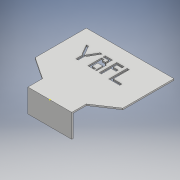
# Autodesk Inventor part: Body Front
Saved by Autodesk Inventor 2018 (Build 220112000, 112)
## iProperties
Created: 2018-04-26
Part Number: Body Front
Material: Generic
Document SubType Name: Modeling
Designer: HP
Density: 1 g/cm^3
Appearance: Default
Author: HP
Autodesk Inventor part; units mm, degrees
ref_plane "YZ Plane" through (0, 0, 0) normal (1, 0, 0) x (0, 1, 0)
ref_plane "XZ Plane" through (0, 0, 0) normal (0, 1, 0) x (-1, 0, 0)
ref_plane "XY Plane" through (0, 0, 0) normal (0, 0, 1) x (1, 0, 0)
sketch "Sketch1" plane through (0, 0, 0) normal (0, 0, 1) x (1, 0, 0)
  line L0 (-30, 0) -> (30, 0)
  line L1 (30, 0) -> (30, 20)
  line L2 (-30, 20) -> (-30, 0)
  line L3 (60, 40) -> (60, 110)
  line L4 (60, 110) -> (-60, 110)
  line L5 (-60, 110) -> (-60, 40)
  line L6 (-60, 40) -> (-30, 20)
  line L7 (30, 20) -> (60, 40)
  point P0 (0, 0)
  dimension "d0" = 60
  dimension "d1" = 20
  dimension "d2" = 120
  dimension "d3" = 70
  constraints: 16 end point, 2 parallel, 1 horizontal, 1 perpendicular
  measures "d0" distance of L2.start L1.end
  measures "d1" distance of L1.end L0.end
  measures "d2" distance of L4.end L3.end
  measures "d3" distance of L3.end L3.start
extrude "Extrusion1" add sketch "Sketch1" along normal blind 2
sketch "Sketch2" plane through (-30, 0, 0) normal (0, -1, 0) x (1, 0, 0)
  line L0 (60, 0) -> (60, 2) projected
  line L1 (60, 0) -> (0, 0)
  line L2 (0, 0) -> (0, -30)
  line L3 (0, -30) -> (60, -30)
  line L4 (60, -30) -> (60, 0)
  point P0 (30, 0)
  dimension "d6" = 60
  dimension "d7" = 30
  constraints: 8 end point, 2 parallel, 1 horizontal, 1 perpendicular
  measures "d6" distance of L3.end L2.end
  measures "d7" distance of L2.end L1.end
extrude "Extrusion2" add sketch "Sketch2" against normal blind 2
sketch "Sketch3" plane through (0, 0, 2) normal (0, 0, 1) x (1, 0, 0)
  line L0 (-37, 90) -> (-29.0967, 76.3111)
  line L1 (-37, 90) -> (-21.1935, 90) construction
  line L2 (-30.5967, 76.3111) -> (-32.0967, 76.3111)
  line L3 (-32.0967, 76.3111) -> (-39.25, 88.701)
  line L4 (-39.25, 88.701) -> (-40, 90)
  line L5 (-40, 90) -> (-37, 90)
  line L6 (-29.0967, 76.3111) -> (-21.1935, 90)
  line L7 (-21.1935, 90) -> (-18.1935, 90)
  line L8 (-18.1935, 90) -> (-26.0967, 76.3111)
  line L9 (-26.0967, 76.3111) -> (-27.5967, 76.3111)
  line L10 (-30.5967, 76.3111) -> (-30.5967, 66.3111)
  line L11 (-30.5967, 66.3111) -> (-27.5967, 66.3111)
  line L12 (-27.5967, 66.3111) -> (-27.5967, 76.3111)
  line L13 (-14.1935, 90) -> (-14.1935, 66.3111)
  line L14 (-14.1935, 90) -> (-4.1935, 90)
  line L15 (-4.1935, 90) -> (-4.1935, 79.933)
  line L16 (-4.1935, 79.933) -> (-2.1935, 79.933)
  line L17 (-2.1935, 79.933) -> (-2.1935, 66.3111)
  line L18 (-2.1935, 66.3111) -> (-14.1935, 66.3111)
  line L19 (-10.757, 87) -> (-10.757, 82.506)
  line L20 (-10.757, 82.506) -> (-6.2868, 82.506)
  line L21 (-6.2868, 82.506) -> (-6.2868, 87)
  line L22 (-6.2868, 87) -> (-10.757, 87)
  line L23 (-10.757, 76.3111) -> (-10.757, 68.4995)
  line L24 (-10.757, 68.4995) -> (-3.7569, 68.4995)
  line L25 (-3.7569, 68.4995) -> (-3.7569, 76.3111)
  line L26 (-3.7569, 76.3111) -> (-10.757, 76.3111)
  line L27 (1.8065, 65.8916) -> (1.8065, 90)
  line L28 (1.8065, 90) -> (11.8065, 90)
  line L29 (11.8065, 90) -> (11.8065, 87)
  line L30 (11.8065, 87) -> (4.8065, 87)
  line L31 (4.8065, 87) -> (4.8065, 82)
  line L32 (4.8065, 82) -> (11.8065, 82)
  line L33 (11.8065, 82) -> (11.8065, 79)
  line L34 (11.8065, 79) -> (4.8065, 79)
  line L35 (4.8065, 79) -> (4.8065, 65.8916)
  line L36 (4.8065, 65.8916) -> (1.8065, 65.8916)
  line L37 (15.8065, 90) -> (15.8065, 64.9111)
  line L38 (15.8065, 64.9111) -> (30.8065, 64.9111)
  line L39 (30.8065, 64.9111) -> (30.8065, 67.9111)
  line L40 (30.8065, 67.9111) -> (18.8065, 67.9111)
  line L41 (18.8065, 67.9111) -> (18.8065, 90)
  line L42 (18.8065, 90) -> (15.8065, 90)
  point P0 (0, 0)
  dimension "d10" = 60
  dimension "d12" = 3
  dimension "d13" = 60
  dimension "d14" = 10
  dimension "d15" = 10
  dimension "d16" = 2
  dimension "d17" = 10
  dimension "d19" = 3
  dimension "d20" = 7
  dimension "d21" = 5
  dimension "d22" = 3
  dimension "d23" = 15
  dimension "d25" = 3
  dimension "d26" = 12
  dimension "d27" = 4
  dimension "d28" = 4
  dimension "d29" = 4
  constraints: 86 end point, 20 perpendicular, 7 vertical, 5 point on line, 4 horizontal, 3 parallel, 1 equal length
  measures "d10" angle of L0 L1
  measures "d12" distance of L1.end L7.end
  measures "d13" angle of L7 L8
  measures "d14" distance of L2.start L10.end
  measures "d15" distance of L13.start L14.end
  measures "d16" distance of L15.end L16.end
  measures "d17" distance of L27.end L28.end
  measures "d19" distance of L28.end L29.end
  measures "d20" distance of L29.end L30.end
  measures "d21" distance of L30.end L31.end
  measures "d22" distance of L32.end L33.end
  measures "d23" distance of L37.end L38.end
  measures "d25" distance of L38.end L39.end
  measures "d26" distance of L39.end L40.end
  measures "d27" distance of L13.start L7.end
  measures "d28" distance between parallel lines of L27 L17
  measures "d29" distance between parallel lines of L37 L33
extrude "Extrusion3" cut sketch "Sketch3" against normal blind 2
sketch "Sketch4" plane through (0, 0, 2) normal (0, 0, 1) x (1, 0, 0)
  point P0 (0, 0)
sketch "Sketch5" plane through (0, 0, 2) normal (0, 0, 1) x (1, 0, 0)
  point P0 (0, 0)
sketch "Sketch6" plane through (0, 0, 2) normal (0, 0, 1) x (1, 0, 0)
  line L0 (-14.1935, 66.3111) -> (-2.1935, 66.3111) projected
  line L1 (-3.7569, 68.4995) -> (-5.7569, 68.4995)
  line L2 (-5.7569, 68.4995) -> (-5.7569, 66.3111)
  line L3 (-5.7569, 66.3111) -> (-3.7569, 66.3111)
  line L4 (-3.7569, 66.3111) -> (-3.7569, 68.4995)
  line L5 (-14.1935, 90) -> (-14.1935, 66.3111) projected
  line L6 (-10.757, 87) -> (-14.1935, 87)
  line L7 (-14.1935, 87) -> (-14.1935, 85)
  line L8 (-14.1935, 85) -> (-10.757, 85)
  line L9 (-10.757, 85) -> (-10.757, 87)
  point P0 (0, 0)
  dimension "d32" = 2
  dimension "d33" = 2
  constraints: 16 end point, 4 parallel, 2 horizontal, 2 perpendicular, 2 point on line
  measures "d32" distance of L3.end L2.end
  measures "d33" distance of L7.end L6.end
extrude "Extrusion4" add sketch "Sketch6" against normal blind 2
sketch "Sketch7" plane through (0, 0, 2) normal (0, 0, 1) x (1, 0, 0)
  point P0 (0, 0)
sketch "Sketch8" plane through (-60, 110, 0) normal (0, 1, 0) x (1, 0, 0)
  line L0 (45, 0) -> (75, 0)
  line L1 (75, 0) -> (75, 30)
  line L2 (75, 30) -> (45, 30)
  line L3 (45, 30) -> (45, 0)
  point P0 (60, 0)
  dimension "d36" = 30
  dimension "d37" = 30
  constraints: 8 end point, 2 parallel, 1 horizontal, 1 perpendicular
  measures "d36" distance of L2.end L1.end
  measures "d37" distance of L1.end L0.end
extrude "Extrusion5" add sketch "Sketch8" against normal blind 2
body "Solid1"
